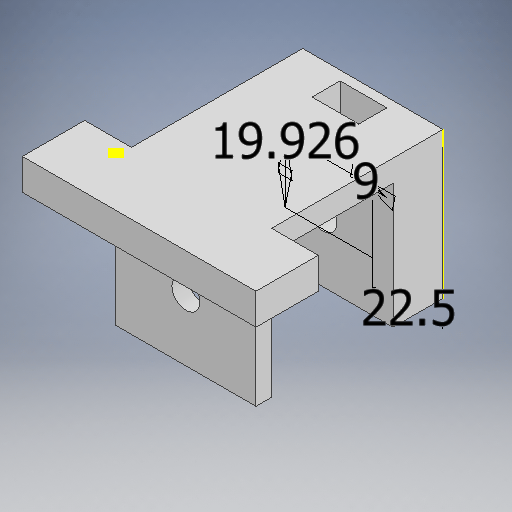
# Autodesk Inventor part: camera_case_bottom_new
Saved by Autodesk Inventor 2025.2 (Build 292293000, 293)
## iProperties
Created: 2025-03-10
Part Number: camera_case_bottom_new
Material: 일반
Document SubType Name: Modeling
Designer: jbhma
Density: 1 g/cm^3
Appearance: 기본값
Author: jbhma
Autodesk Inventor part; units mm, degrees
ref_plane "YZ Plane" through (0, 0, 0) normal (1, 0, 0) x (0, 1, 0)
ref_plane "XZ Plane" through (0, 0, 0) normal (0, 1, 0) x (-1, 0, 0)
ref_plane "XY Plane" through (0, 0, 0) normal (0, 0, 1) x (1, 0, 0)
sketch "스케치17" plane through (0, 0, 0) normal (1, 0, 0) x (0, 1, 0)
  line L0 (0, 0) -> (40, 0)
  line L1 (40, 0) -> (40, -5)
  line L2 (40, -5) -> (0, -5)
  line L3 (0, -5) -> (0, 0)
  line L4 (40, 0) -> (47, 0)
  line L5 (47, 0) -> (47, -60)
  line L6 (47, -60) -> (40, -60)
  line L7 (40, -60) -> (40, 0)
  line L8 (40, -60) -> (0, -60)
  line L9 (0, -60) -> (0, -44)
  line L10 (0, -44) -> (40, -44)
  line L11 (40, -44) -> (40, -60)
  dimension "d51" = 40
  dimension "d52" = 5
  dimension "d53" = 7
  dimension "d54" = 60
  dimension "d55" = 40
  dimension "d56" = 16
  constraints: 24 end point, 6 parallel, 3 horizontal, 3 perpendicular
  measures "d51" distance of L1.end L2.end
  measures "d52" distance of L0.end L1.end
  measures "d53" distance of L5.end L6.end
  measures "d54" distance of L4.end L5.end
  measures "d55" distance of L9.end L10.end
  measures "d56" distance of L8.end L9.end
extrude "돌출13" add sketch "스케치17" along normal blind 45
sketch "스케치18" plane through (0, 0, 0) normal (0, 0, 1) x (1, 0, 0)
  circle A0 centre (22.5, 19.926) radius 4.5
  line L0 (0, 0) -> (45, 0) projected
  line L1 (0, 47) -> (0, 0) projected
  dimension "d59" = 9
  dimension "d60" = 19.926
  dimension "d64" = 22.5
  constraints: 1 centre point
  measures "d59" diameter of A0
  measures "d60" distance from line of L0 A0.centre
  measures "d64" distance from line of A0.centre L1
sketch "스케치19" plane through (0, 0, -60) normal (0, 0, -1) x (-1, 0, 0)
  circle A0 centre (-22.5, 19.926) radius 4.5
  line L0 (0, 0) -> (-45, 0) projected
  line L1 (-45, 0) -> (-45, 47) projected
  point P0 (-22.5, 0)
  dimension "d61" = 9
  dimension "d62" = 19.926
  dimension "d63" = 22.5
  constraints: 1 centre point, 1 midpoint
  measures "d61" diameter of A0
  measures "d62" distance of A0.centre point (-22.5, 0)
  measures "d63" distance from line of A0.centre L1
extrude "돌출14" cut sketch "스케치18" against normal blind 100
sketch "스케치20" plane through (0, 47, 0) normal (0, 1, 0) x (1, 0, 0)
  point P0 (0, 0)
sketch "스케치21" plane through (0, 47, 0) normal (0, 1, 0) x (1, 0, 0)
  line L0 (15, 57) -> (30, 57)
  line L1 (30, 57) -> (30, 48)
  line L2 (30, 48) -> (15, 48)
  line L3 (15, 48) -> (15, 57)
  line L4 (0, 60) -> (0, 0) projected
  line L5 (0, 60) -> (45, 60) projected
  point P0 (15, 52.5)
  point P1 (22.5, 57)
  dimension "d67" = 15
  dimension "d68" = 9
  dimension "d69" = 15
  dimension "d70" = 3
  constraints: 8 end point, 2 midpoint, 2 parallel, 1 horizontal, 1 perpendicular
  measures "d67" distance of L1.end L2.end
  measures "d68" distance of L0.end L1.end
  measures "d69" distance from line of point (15, 52.5) L4
  measures "d70" distance from line of point (22.5, 57) L5
extrude "돌출15" cut sketch "스케치21" against normal blind 13
sketch "스케치22" plane through (0, 0, 0) normal (0, 0, 1) x (1, 0, 0)
  line L0 (0, 47) -> (45, 47)
  line L1 (45, 47) -> (45, 37)
  line L2 (45, 37) -> (0, 37)
  line L3 (0, 37) -> (0, 47)
  point P0 (0, 0)
  constraints: 8 end point, 2 parallel, 1 horizontal, 1 perpendicular
extrude "돌출16" add sketch "스케치22" along normal blind 15
sketch "스케치23" plane through (45, 0, 0) normal (1, 0, 0) x (0, 0, -1)
  line L0 (-15, 47) -> (5, 47)
  line L1 (5, 47) -> (5, 37)
  line L2 (5, 37) -> (-15, 37)
  line L3 (-15, 37) -> (-15, 47)
  point P0 (0, 0)
  constraints: 8 end point, 2 parallel, 1 horizontal, 1 perpendicular
sketch "스케치24" plane through (0, 0, 0) normal (-1, 0, 0) x (0, 0, 1)
  line L0 (15, 47) -> (-5, 47)
  line L1 (-5, 47) -> (-5, 37)
  line L2 (-5, 37) -> (15, 37)
  line L3 (15, 37) -> (15, 47)
  point P0 (0, 0)
  constraints: 8 end point, 2 parallel, 1 horizontal, 1 perpendicular
extrude "돌출17" add sketch "스케치24" along normal blind 15
extrude "돌출18" add sketch "스케치23" along normal blind 15
